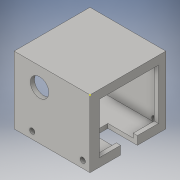
# Autodesk Inventor part: Chasis_rework
Saved by Autodesk Inventor 2016 (Build 200138000, 138)
## iProperties
Created: 2016-03-17
Part Number: Chasis_rework
Material: Generic
Document SubType Name: Modeling
Designer: torti_000
Density: 1 g/cm^3
Appearance: Default
Author: torti_000
Autodesk Inventor part; units mm, degrees
ref_plane "YZ Plane" through (0, 0, 0) normal (1, 0, 0) x (0, 1, 0)
ref_plane "XZ Plane" through (0, 0, 0) normal (0, 1, 0) x (-1, 0, 0)
ref_plane "XY Plane" through (0, 0, 0) normal (0, 0, 1) x (1, 0, 0)
sketch "Sketch1" plane through (0, 0, 0) normal (0, 1, 0) x (-1, 0, 0)
  line L0 (114.3, 0) -> (114.3, -114.3)
  line L1 (114.3, -114.3) -> (0, -114.3)
  line L2 (25.4, -71.4495) -> (0, -71.4495)
  line L3 (25.4, -46.0495) -> (0, -46.0495)
  line L4 (0, -114.3) -> (0, -71.4495)
  line L5 (114.3, 0) -> (0, 0)
  line L6 (0, 0) -> (0, -46.0495)
  line L7 (25.4, -71.4495) -> (44.45, -71.4495)
  line L8 (44.45, -71.4495) -> (44.45, -46.0495)
  line L9 (44.45, -46.0495) -> (25.4, -46.0495)
  constraints: 20 end point, 4 perpendicular, 2 horizontal, 1 parallel
extrude "Extrusion1" add sketch "Sketch1" along normal blind 6.35
sketch "Sketch2" plane through (0, 6.35, 0) normal (0, 1, 0) x (1, 0, 0)
  line L0 (-114.3, 0) -> (0, 0) projected
  line L1 (-114.3, 0) -> (-114.3, 6.35)
  line L2 (-114.3, 114.3) -> (-114.3, 0) projected
  line L3 (-114.3, 6.35) -> (0, 6.35)
  line L4 (0, 0) -> (0, 46.0495) projected
  line L5 (0, 0) -> (-114.3, 0)
  line L6 (0, 114.3) -> (-114.3, 114.3) projected
  line L7 (0, 114.3) -> (0, 107.95)
  line L8 (0, 114.3) -> (0, 71.4495) projected
  line L9 (0, 107.95) -> (-114.3, 107.95)
  line L10 (-114.3, 114.3) -> (0, 114.3)
  constraints: 12 end point, 4 point on line, 2 collinear, 2 perpendicular
extrude "Extrusion2" add sketch "Sketch2" along normal blind 88.9
sketch "Sketch3" plane through (0, 95.25, 0) normal (0, 1, 0) x (1, 0, 0)
  line L0 (-114.3, 6.35) -> (-114.3, 0) projected
  line L1 (0, 114.3) -> (-114.3, 114.3) projected
  line L2 (-114.3, 0) -> (0, 0)
  line L3 (0, 0) -> (0, 114.3)
  line L4 (0, 114.3) -> (-114.3, 114.3)
  line L5 (-114.3, 114.3) -> (-114.3, 0)
  point P0 (0, 0)
  constraints: 8 end point, 2 parallel, 1 horizontal, 1 perpendicular
extrude "Extrusion3" add sketch "Sketch3" along normal blind 6.35
sketch "Sketch4" plane through (0, 6.35, 0) normal (0, 1, 0) x (1, 0, 0)
  line L0 (0, 6.35) -> (0, 46.0495) projected
  line L1 (0, 107.95) -> (-114.3, 107.95) projected
  line L2 (0, 6.35) -> (0, 107.95)
  line L3 (0, 6.35) -> (-6.35, 6.35)
  line L4 (-114.3, 6.35) -> (0, 6.35) projected
  line L5 (-6.35, 6.35) -> (-6.35, 107.95)
  line L6 (0, 71.4495) -> (0, 107.95) projected
  line L7 (0, 107.95) -> (-6.35, 107.95)
  point P0 (0, 0)
  dimension "d13" = 6.35
  constraints: 8 end point, 2 perpendicular, 2 point on line, 1 collinear
  measures "d13" distance of L0.start L3.end
extrude "Extrusion4" add sketch "Sketch4" along normal blind 88.9
sketch "Sketch5" plane through (0, 0, 0) normal (1, 0, 0) x (0, 0, -1)
  line L0 (46.0495, 6.35) -> (71.4495, 6.35) projected
  line L1 (46.0495, 6.35) -> (71.4495, 6.35)
  line L2 (71.4495, 6.35) -> (71.4495, 12.7)
  line L3 (46.0495, 12.7) -> (46.0495, 6.35)
  line L4 (46.0495, 12.7) -> (14.2995, 12.7)
  line L5 (71.4495, 12.7) -> (103.1995, 12.7)
  line L6 (103.1995, 12.7) -> (103.1995, 88.9)
  line L7 (107.95, 95.25) -> (6.35, 95.25) projected
  line L8 (103.1995, 88.9) -> (14.2995, 88.9)
  line L9 (14.2995, 88.9) -> (14.2995, 12.7)
  point P0 (0, 0)
  constraints: 16 end point, 4 horizontal, 3 perpendicular, 1 parallel
extrude "Extrusion5" cut sketch "Sketch5" against normal blind 6.35
sketch "Sketch6" plane through (0, 6.35, 0) normal (0, 1, 0) x (1, 0, 0)
  line L0 (-114.3, 107.95) -> (-114.3, 6.35) projected
  line L1 (-114.3, 6.35) -> (-114.3, 107.95)
  line L2 (-114.3, 107.95) -> (-107.95, 107.95)
  line L3 (-107.95, 107.95) -> (-107.95, 6.35)
  line L4 (-107.95, 6.35) -> (-114.3, 6.35)
  point P0 (0, 0)
  constraints: 8 end point, 2 equal length, 2 perpendicular
extrude "Extrusion6" add sketch "Sketch6" along normal blind 88.9
sketch "Sketch7" plane through (-114.3, 0, -114.3) normal (-1, 0, 0) x (0, 0, 1)
  line L0 (100.0005, 88.9) -> (11.1005, 88.9) projected
  line L1 (100.0005, 88.9) -> (100.0005, 12.7) projected
  line L2 (11.1005, 88.9) -> (100.0005, 88.9)
  line L3 (100.0005, 88.9) -> (100.0005, 12.7)
  line L4 (100.0005, 12.7) -> (11.1005, 12.7)
  line L5 (11.1005, 12.7) -> (11.1005, 88.9)
  point P0 (114.3, 0)
  constraints: 8 end point, 2 parallel, 1 horizontal, 1 perpendicular
extrude "Extrusion7" cut sketch "Sketch7" against normal blind 6.35
sketch "Sketch8" plane through (0, 0, -114.3) normal (0, 0, -1) x (-1, 0, 0)
  line L0 (114.3, 0) -> (0, 0) projected
  line L1 (6.35, 6.35) -> (107.95, 6.35) projected
  circle A0 centre (10.8401, 10.8401) radius 4.4901
  constraints: 1 centre point, 1 tangent
hole "Hole1" at (-10.8401, 10.8401, -114.3) direction (0, 0, 1) diameter 7.9375 end through all
sketch "Sketch9" plane through (0, 0, -114.3) normal (0, 0, -1) x (-1, 0, 0)
  circle A0 centre (10.8401, 10.8401) radius 3.9687 projected
  circle A1 centre (87.0401, 10.8401) radius 3.9688
  point P0 (0, 0)
  constraints: 1 centre point
hole "Hole2" at (-87.0401, 10.8401, -114.3) direction (0, 0, 1) diameter 7.9375 end through all
sketch "Sketch10" plane through (0, 0, -114.3) normal (0, 0, -1) x (-1, 0, 0)
  circle A0 centre (87.0401, 10.8401) radius 3.9687 projected
  line L0 (87.0401, 10.8401) -> (150.5401, 10.8401) construction
  circle A1 centre (76.0135, 73.3754) radius 14
  point P0 (0, 0)
  constraints: 2 end point, 1 centre point, 1 horizontal
hole "Hole3" at (-76.0135, 73.3754, -114.3) direction (0, 0, 1) diameter 28 end through all
sketch "Sketch11" plane through (0, 101.6, 0) normal (0, 1, 0) x (1, 0, 0)
  point P0 (0, 0)
body "Solid1"
